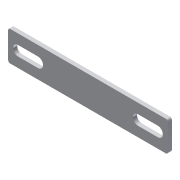
# Autodesk Inventor part: PS20013
Saved by Autodesk Inventor 2014 (Build 180170000, 170)
## iProperties
Category: NS
Created: 2012-04-24
Part Number: PS20013
Material: UHMW, White
Document SubType Name: Modeling
Designer: ERF
Mass: 1.99257 g
Surface Area: 26.3914 cm^2
Volume: 2.11976 cm^3
Density: 0.94 g/cm^3
Stock Number: PS20013
Description: Universal Spindle Mount strap
Vendor: ProkTech
Project: Shapeoko
Appearance: Smooth - White
User Status: F
Authority: PER BARRY PROCK 9-16-13
Author: ERF
Title: Spindle Strap
Subject: Clamping
Comments: Fusion
Autodesk Inventor part; units mm, degrees
ref_plane "YZ Plane" through (0, 0, 0) normal (1, 0, 0) x (0, 1, 0)
ref_plane "XZ Plane" through (0, 0, 0) normal (0, 1, 0) x (-1, 0, 0)
ref_plane "XY Plane" through (0, 0, 0) normal (0, 0, 1) x (1, 0, 0)
sketch "Sketch1" plane through (0, 0, 0) normal (0, 0, 1) x (1, 0, 0)
  line L0 (-40, 7.5) -> (40, 7.5)
  line L1 (40, 7.5) -> (40, -7.5)
  line L2 (40, -7.5) -> (-40, -7.5)
  line L3 (-40, -7.5) -> (-40, 7.5)
  point P0 (0, 0)
  dimension "d0" = 80
  dimension "d1" = 15
  dimension "d2" = 40
  dimension "d3" = 7.5
  constraints: 8 end point, 2 parallel, 1 horizontal, 1 perpendicular
  measures "d0" distance of L1.end L2.end
  measures "d1" distance of L0.end L1.end
  measures "d2" distance from line of point (0, 0) L3
  measures "d3" distance from line of L0 point (0, 0)
extrude "Extrusion1" add sketch "Sketch1" along normal blind 2
sketch "Sketch2" plane through (0, 0, 2) normal (0, 0, 1) x (1, 0, 0)
  line L0 (-40, 7.5) -> (40, 7.5) projected
  line L1 (-40, -7.5) -> (-40, 7.5) projected
  arc A0 (-35, 2.5) -> (-35, -2.5) centre (-35, 0) ccw
  arc A1 (-25, -2.5) -> (-25, 2.5) centre (-25, 0) ccw
  line L2 (-35, 2.5) -> (-25, 2.5)
  line L3 (-25, -2.5) -> (-35, -2.5)
  arc A2 (25, 2.5) -> (25, -2.5) centre (25, 0) ccw
  arc A3 (35, -2.5) -> (35, 2.5) centre (35, 0) ccw
  line L4 (25, 2.5) -> (35, 2.5)
  line L5 (35, -2.5) -> (25, -2.5)
  point P0 (0, 0)
  dimension "d6" = 5
  dimension "d7" = 5
  dimension "d8" = 10
  dimension "d9" = 5
  dimension "d10" = 7.5
  dimension "d11" = 7.5
  dimension "d12" = 5
  dimension "d15" = 60
  constraints: 8 end point, 8 point on circle, 4 centre point, 3 tangent, 1 horizontal, 10 other
  measures "d6" diameter of A0
  measures "d7" diameter of A1
  measures "d8" distance of A0.centre A1.centre
  measures "d9" distance from line of L1 A0.centre
  measures "d10" distance from line of L0 A0.centre
  measures "d11" distance from line of L0 A1.centre
  measures "d12" distance of L3.end L2.start
  measures "d15" distance of A0.centre A2.centre
extrude "Extrusion2" cut sketch "Sketch2" against normal through all
fillet "Fillet1" radius 1 4 edges at (-40, 7.5, 1) (-40, -7.5, 1) (40, -7.5, 1) (40, 7.5, 1)
equation "\"d2\" = 0.5 * d0"
equation "\"d3\" = 0.5 * d1"
body "Solid1"
